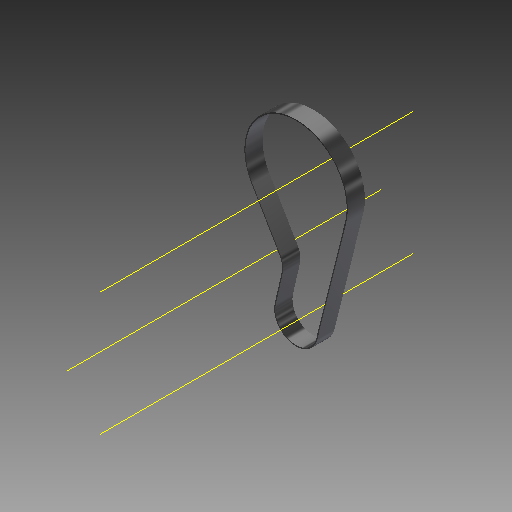
# Autodesk Inventor part: Synchronous Belt
Saved by Autodesk Inventor 2019.4 (Build 234330000, 330)
## iProperties
Created: 2019-11-30
Part Number: Synchronous Belt
Material: Rubber
Document SubType Name: Modeling
Designer: admin
Density: 0.93 g/cm^3
Appearance: Rubber - Black - Version 1.1
Mass: 6.7704 g
Surface Area: 154.7 cm^2
Volume: 7.28 cm^3
CustomPartVersion: 1
Author: admin
Autodesk Inventor part; units mm, degrees
ref_plane "YZ Plane" through (0, 0, 0) normal (1, 0, 0) x (0, 1, 0)
ref_plane "XZ Plane" through (0, 0, 0) normal (0, 1, 0) x (-1, 0, 0)
ref_plane "XY Plane" through (0, 0, 0) normal (0, 0, 1) x (1, 0, 0)
sketch "Sketch Path" plane through (0, 0, 0) normal (0, 0, 1) x (1, 0, 0)
  arc A0 (46.3191, -11.5873) -> (-41.2118, -24.1104) centre (0, 0) ccw
  arc A1 (-19.3819, -110.2804) -> (19.2996, -119.5947) centre (0, -114.7666) ccw
  arc A2 (-12.8487, -82.0549) -> (-14.7938, -69.2665) centre (-29.9048, -78.107) ccw
  line L0 (-14.7938, -69.2665) -> (-41.2118, -24.1104)
  line L1 (46.3191, -11.5873) -> (19.2996, -119.5947)
  line L2 (-19.3819, -110.2804) -> (-12.8487, -82.0549)
  constraints: 6 end point, 4 point on circle, 2 centre point, 3 other
ref_plane "Cross Section Plane" through (-41.2118, -24.1104, 0) normal (0.5049679, -0.8631381, 0) x (0, 0, 1)
ref_plane "Work Plane2" through (0, 0, 0) normal (-1, 0, 0) x (0, 0, 1)
ref_plane "Work Plane3" through (0, -114.7666, 0) normal (0.3369317, 0.9415291, 0) x (0, 0, 1)
ref_plane "Work Plane6" through (-29.9048, -78.107, 0) normal (0.1785215, 0.983936, 0) x (0, 0, 1)
sketch "Cross Section" plane through (-41.2118, -24.1104, 0) normal (0.5049679, -0.8631381, 0) x (0, 0, 1)
  line L0 (-8, 0.5) -> (8, 0.5)
  line L1 (8, 0.5) -> (8, -0.5)
  line L2 (8, -0.5) -> (-8, -0.5)
  line L3 (-8, -0.5) -> (-8, 0.5)
  line L4 (-8, 0) -> (8, 0) construction
  point P0 (0, 0)
  point P1 (0, 0)
  dimension "d0" = 16
  dimension "d4" = 0.5
  dimension "d5" = 0.5
  constraints: 10 end point, 3 midpoint, 2 parallel, 1 coincident, 1 horizontal, 1 perpendicular, 1 other
  measures "d0" distance between parallel lines of L1 L3
  measures "d4" distance between parallel lines of L2 L4
  measures "d5" distance between parallel lines of L4 L0
sweep "Belt" add profiles "Cross Section" path "Sketch Path" path curves L2 A2 L0 A0 L1 A1
equation "\"d0\" = da_B"
equation "\"d4\" = da_a"
equation "\"d5\" = da_a2"
equation "\"da_B\" = 16"
equation "\"da_pb\" = 5"
equation "\"da_L\" = 455"
equation "\"da_a\" = 0.5"
equation "\"da_S\" = 2.65"
equation "\"da_Beta\" = 20deg"
equation "\"da_Ht\" = 1.2"
equation "\"da_H\" = 2.2"
equation "\"da_a2\" = 0.5"
body "Solid1"
